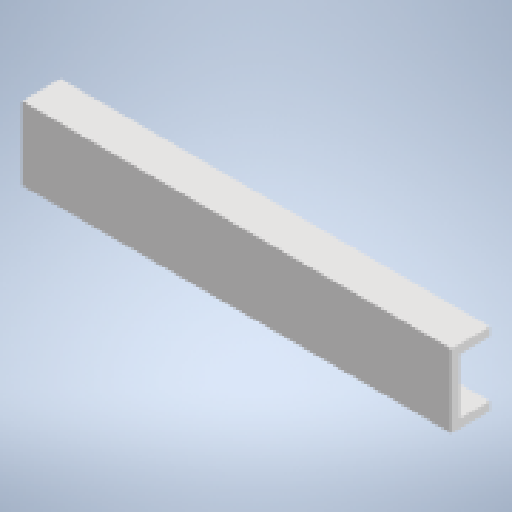
# Autodesk Inventor part: Channel
Saved by Autodesk Inventor 2024.2 (Build 282272000, 272)
## iProperties
Created: 2024-01-22
Part Number: Channel
Material: Generic
Document SubType Name: Modeling
Designer: Felix
Density: 1 g/cm^3
Appearance: Default
Author: Felix
Autodesk Inventor part; units mm, degrees
ref_plane "YZ Plane" through (0, 0, 0) normal (1, 0, 0) x (0, 1, 0)
ref_plane "XZ Plane" through (0, 0, 0) normal (0, 1, 0) x (-1, 0, 0)
ref_plane "XY Plane" through (0, 0, 0) normal (0, 0, 1) x (1, 0, 0)
sketch "Sketch1" plane through (0, 0, 0) normal (1, 0, 0) x (0, 1, 0)
  line L0 (9, 8.5) -> (0, 8.5)
  line L1 (0, 8.5) -> (0, -8.5)
  line L2 (0, -8.5) -> (9, -8.5)
  line L3 (9, -8.5) -> (9, -6.5)
  line L4 (9, 6.5) -> (2, 6.5)
  line L5 (2, 6.5) -> (2, -6.5)
  line L6 (2, -6.5) -> (9, -6.5)
  line L7 (9, -6.5) -> (9, 6.5) construction
  line L8 (9, 6.5) -> (9, 8.5)
  line L9 (9, -6.5) -> (9, 6.5) construction
  point P0 (0, 0)
  point P1 (0, 0)
  dimension "d0" = 9
  dimension "d1" = 17
  dimension "d3" = 13
  dimension "d4" = 2
  dimension "d5" = 2
  dimension "d6" = 2
  constraints: 20 end point, 6 parallel, 2 horizontal, 2 perpendicular, 1 coincident, 1 midpoint
  measures "d0" distance of L2.end L1.end
  measures "d1" distance of L1.end L0.end
  measures "d3" distance of L4.end L5.end
  measures "d4" distance between parallel lines of L1 L5
  measures "d5" distance between parallel lines of L0 L4
  measures "d6" distance between parallel lines of L2 L6
extrude "Extrusion1" add sketch "Sketch1" along normal blind 100
equation "\"d5\" = d6"
body "Solid1"
